Autodesk Inventor part; units mm, degrees
(part 3 of 3)
  line L1861 (14.3835, -12.5591) -> (14.4054, -12.4772)
  line L1862 (17.1782, -13.4855) -> (17.1805, -13.4518)
  line L1863 (17.0231, -13.6469) -> (17.0963, -13.6273)
  line L1864 (17.0963, -13.6273) -> (17.1562, -13.5674)
  line L1865 (17.1562, -13.5674) -> (17.1782, -13.4855)
  line L1866 (6.3458, -17.4083) -> (6.4277, -17.4302)
  line L1867 (6.4277, -17.4302) -> (6.5095, -17.4083)
  line L1868 (6.5095, -17.4083) -> (6.5695, -17.3484)
  line L1869 (6.5695, -17.3484) -> (6.5731, -17.2918)
  line L1870 (1.5112, -17.3523) -> (1.5566, -17.4083)
  line L1871 (1.5566, -17.4083) -> (1.6384, -17.4302)
  line L1872 (1.6384, -17.4302) -> (1.7203, -17.4083)
  line L1873 (1.7203, -17.4083) -> (1.7976, -17.3523)
  line L1874 (-4.3089, -17.3184) -> (-4.3009, -17.3484)
  line L1875 (-4.3009, -17.3484) -> (-4.241, -17.4083)
  line L1876 (-4.241, -17.4083) -> (-4.1591, -17.4302)
  line L1877 (-4.1591, -17.4302) -> (-4.0772, -17.4083)
  line L1878 (-4.0772, -17.4083) -> (-4.049, -17.3801)
  line L1879 (-0.2705, -17.3523) -> (-0.2079, -17.4083)
  line L1880 (-0.2079, -17.4083) -> (-0.126, -17.4302)
  line L1881 (-0.126, -17.4302) -> (-0.0442, -17.4083)
  line L1882 (-0.0442, -17.4083) -> (0.0159, -17.3523)
  line L1883 (-6.0807, -15.5268) -> (-6.0653, -15.5839)
  line L1884 (-6.0653, -15.5839) -> (-6.0054, -15.6438)
  line L1885 (-6.0054, -15.6438) -> (-5.9235, -15.6658)
  line L1886 (-5.9235, -15.6658) -> (-5.8417, -15.6438)
  line L1887 (-5.8417, -15.6438) -> (-5.8234, -15.6256)
  line L1888 (-9.1183, -14.7466) -> (-9.0901, -14.8277)
  line L1889 (-9.0901, -14.8277) -> (-9.0302, -14.8876)
  line L1890 (-9.0302, -14.8876) -> (-8.9483, -14.9096)
  line L1891 (-8.9483, -14.9096) -> (-8.8703, -14.8897)
  line L1892 (-11.8848, -14.7458) -> (-11.8629, -14.8277)
  line L1893 (-11.8629, -14.8277) -> (-11.8029, -14.8876)
  line L1894 (-11.8029, -14.8876) -> (-11.721, -14.9096)
  line L1895 (-11.721, -14.9096) -> (-11.6701, -14.8897)
  line L1896 (-13.6492, -15.7541) -> (-13.6273, -15.836)
  line L1897 (-13.6273, -15.836) -> (-13.5674, -15.8959)
  line L1898 (-13.5674, -15.8959) -> (-13.4855, -15.9178)
  line L1899 (-13.4855, -15.9178) -> (-13.4518, -15.9078)
  line L1900 (-15.1443, -17.1424) -> (-15.1397, -17.2223)
  line L1901 (-15.1397, -17.2223) -> (-15.0798, -17.2823)
  line L1902 (-15.0798, -17.2823) -> (-14.9979, -17.3042)
  line L1903 (-17.435, -14.5971) -> (-17.4302, -14.6198)
  line L1904 (-17.4302, -14.6198) -> (-17.4083, -14.7017)
  line L1905 (-17.4083, -14.7017) -> (-17.3484, -14.7616)
  line L1906 (-17.3484, -14.7616) -> (-17.2747, -14.7813)
  line L1907 (-15.6533, -13.1972) -> (-15.6658, -13.2334)
  line L1908 (-15.6658, -13.2334) -> (-15.6438, -13.3153)
  line L1909 (-15.6438, -13.3153) -> (-15.5839, -13.3752)
  line L1910 (-15.5839, -13.3752) -> (-15.502, -13.3972)
  line L1911 (-15.1443, -11.4156) -> (-15.1616, -11.469)
  line L1912 (-15.1616, -11.469) -> (-15.1397, -11.5509)
  line L1913 (-15.1397, -11.5509) -> (-15.0798, -11.6108)
  line L1914 (-15.0798, -11.6108) -> (-14.9979, -11.6327)
  line L1915 (-14.8897, -8.6158) -> (-14.9096, -8.6963)
  line L1916 (-14.9096, -8.6963) -> (-14.8876, -8.7781)
  line L1917 (-14.8876, -8.7781) -> (-14.8277, -8.8381)
  line L1918 (-14.8277, -8.8381) -> (-14.7466, -8.8638)
  line L1919 (-15.6275, -6.0774) -> (-15.6438, -6.0937)
  line L1920 (-15.6438, -6.0937) -> (-15.6658, -6.1756)
  line L1921 (-15.6658, -6.1756) -> (-15.6438, -6.2575)
  line L1922 (-15.6438, -6.2575) -> (-15.5839, -6.3174)
  line L1923 (-15.5839, -6.3174) -> (-15.5101, -6.3185)
  line L1924 (-17.3801, -4.049) -> (-17.4083, -4.0772)
  line L1925 (-17.4083, -4.0772) -> (-17.4302, -4.1591)
  line L1926 (-17.4302, -4.1591) -> (-17.4083, -4.241)
  line L1927 (-17.4083, -4.241) -> (-17.3484, -4.3009)
  line L1928 (-17.3484, -4.3009) -> (-17.3184, -4.3089)
  line L1929 (-17.3523, -1.5112) -> (-17.4083, -1.5566)
  line L1930 (-17.4083, -1.5566) -> (-17.4302, -1.6384)
  line L1931 (-17.4302, -1.6384) -> (-17.4083, -1.7203)
  line L1932 (-17.4083, -1.7203) -> (-17.3523, -1.7976)
  line L1933 (-17.3523, 1.034) -> (-17.4083, 0.9641)
  line L1934 (-17.4083, 0.9641) -> (-17.4302, 0.8822)
  line L1935 (-17.4302, 0.8822) -> (-17.4083, 0.8004)
  line L1936 (-17.4083, 0.8004) -> (-17.3523, 0.7476)
  line L1937 (-17.3223, 3.8037) -> (-17.3484, 3.7968)
  line L1938 (-17.3484, 3.7968) -> (-17.4083, 3.7368)
  line L1939 (-17.4083, 3.7368) -> (-17.4302, 3.6549)
  line L1940 (-17.4302, 3.6549) -> (-17.4083, 3.5731)
  line L1941 (-17.4083, 3.5731) -> (-17.3762, 3.541)
  line L1942 (-17.2918, 6.8276) -> (-17.3484, 6.8215)
  line L1943 (-17.3484, 6.8215) -> (-17.4083, 6.7616)
  line L1944 (-17.4083, 6.7616) -> (-17.4302, 6.6797)
  line L1945 (-17.4302, 6.6797) -> (-17.4083, 6.5979)
  line L1946 (-17.2918, 9.3729) -> (-17.3484, 9.3422)
  line L1947 (-17.3484, 9.3422) -> (-17.4083, 9.2823)
  line L1948 (-17.4083, 9.2823) -> (-17.4302, 9.2004)
  line L1949 (-17.4302, 9.2004) -> (-17.4117, 9.1311)
  line L1950 (-17.2824, 11.6285) -> (-17.3484, 11.6108)
  line L1951 (-17.3484, 11.6108) -> (-17.4083, 11.5509)
  line L1952 (-17.4083, 11.5509) -> (-17.4302, 11.469)
  line L1953 (-17.4302, 11.469) -> (-17.435, 11.4156)
  line L1954 (-17.0963, 12.8711) -> (-17.1562, 12.8112)
  line L1955 (-15.7541, 13.1451) -> (-15.836, 13.1232)
  line L1956 (-15.836, 13.1232) -> (-15.8959, 13.0632)
  line L1957 (-15.8959, 13.0632) -> (-15.9178, 12.9814)
  line L1958 (-15.9178, 12.9814) -> (-15.9078, 12.9427)
  line L1959 (-13.9608, 17.435) -> (-13.9896, 17.4302)
  line L1960 (-14.0715, 17.4083) -> (-14.1314, 17.3484)
  line L1961 (-12.8112, 17.4083) -> (-12.8711, 17.3484)
  line L1962 (-12.8711, 17.3484) -> (-12.8896, 17.2793)
  line L1963 (-16.2927, 5.5739) -> (-16.3401, 5.5612)
  line L1964 (-16.3401, 5.5612) -> (-16.4, 5.5013)
  line L1965 (-16.4, 5.5013) -> (-16.422, 5.4194)
  line L1966 (-16.422, 5.4194) -> (-16.4, 5.3375)
  line L1967 (-16.4, 5.3375) -> (-16.3795, 5.317)
  line L1968 (-16.01, 11.8838) -> (-16.088, 11.8629)
  line L1969 (-16.088, 11.8629) -> (-16.148, 11.8029)
  line L1970 (-16.148, 11.8029) -> (-16.1699, 11.721)
  line L1971 (-16.1699, 11.721) -> (-16.1624, 11.6701)
  line L1972 (-5.307, 13.9989) -> (-5.3375, 14.0054)
  line L1973 (-5.3375, 14.0054) -> (-5.4194, 14.0273)
  line L1974 (-5.4194, 14.0273) -> (-5.5013, 14.0054)
  line L1975 (-5.5013, 14.0054) -> (-5.5612, 13.9455)
  line L1976 (-5.5612, 13.9455) -> (-5.5789, 13.8796)
  line L1977 (1.034, 17.3523) -> (0.9641, 17.4083)
  line L1978 (0.9641, 17.4083) -> (0.8822, 17.4302)
  line L1979 (0.8822, 17.4302) -> (0.8004, 17.4083)
  line L1980 (0.8004, 17.4083) -> (0.7476, 17.3523)
  line L1981 (7.5912, 16.5282) -> (7.5777, 16.5922)
  line L1982 (7.5777, 16.5922) -> (7.5178, 16.6521)
  line L1983 (7.5178, 16.6521) -> (7.4359, 16.674)
  line L1984 (7.4359, 16.674) -> (7.3541, 16.6521)
  line L1985 (12.4331, 11.7368) -> (12.3512, 11.7588)
  line L1986 (12.3512, 11.7588) -> (12.3175, 11.7497)
  line L1987 (12.5032, 11.5513) -> (12.515, 11.595)
  line L1988 (15.4137, 10.4607) -> (15.3918, 10.5426)
  line L1989 (15.3918, 10.5426) -> (15.3318, 10.6025)
  line L1990 (15.3318, 10.6025) -> (15.25, 10.6245)
  line L1991 (15.3988, 10.3975) -> (15.4137, 10.4607)
  line L1992 (14.4054, 9.7045) -> (14.3835, 9.7864)
  line L1993 (14.3835, 9.7864) -> (14.3236, 9.8463)
  line L1994 (14.3236, 9.8463) -> (14.2375, 9.8819)
  line L1995 (14.3807, 9.6339) -> (14.4054, 9.7045)
  line L1996 (14.1534, 3.6549) -> (14.1314, 3.7368)
  line L1997 (14.1314, 3.7368) -> (14.0715, 3.7968)
  line L1998 (14.0715, 3.7968) -> (14.0202, 3.8105)
  line L1999 (14.0926, 3.5343) -> (14.1314, 3.5731)
  line L2000 (14.1314, 3.5731) -> (14.1534, 3.6549)
  line L2001 (16.1699, -0.6302) -> (16.148, -0.5483)
  line L2002 (16.148, -0.5483) -> (16.0797, -0.4931)
  line L2003 (16.0797, -0.7795) -> (16.148, -0.712)
  line L2004 (16.148, -0.712) -> (16.1699, -0.6302)
  line L2005 (13.6492, -5.9235) -> (13.6273, -5.8417)
  line L2006 (13.6273, -5.8417) -> (13.6171, -5.816)
  line L2007 (13.4947, -6.0848) -> (13.5674, -6.0653)
  line L2008 (13.5674, -6.0653) -> (13.6273, -6.0054)
  line L2009 (13.6273, -6.0054) -> (13.6492, -5.9235)
  line L2010 (14.1534, -7.9401) -> (14.1262, -7.8522)
  line L2011 (13.983, -8.1002) -> (14.0715, -8.0819)
  line L2012 (14.0715, -8.0819) -> (14.1314, -8.0219)
  line L2013 (14.1314, -8.0219) -> (14.1534, -7.9401)
  line L2014 (4.6778, -14.3539) -> (4.7074, -14.3835)
  line L2015 (4.7074, -14.3835) -> (4.7892, -14.4054)
  line L2016 (4.7892, -14.4054) -> (4.8711, -14.3835)
  line L2017 (4.8711, -14.3835) -> (4.9311, -14.3236)
  line L2018 (4.9311, -14.3236) -> (4.9466, -14.2655)
  line L2019 (-1.034, -15.3161) -> (-0.9641, -15.3918)
  line L2020 (-0.9641, -15.3918) -> (-0.8822, -15.4137)
  line L2021 (-0.8822, -15.4137) -> (-0.8004, -15.3918)
  line L2022 (-0.8004, -15.3918) -> (-0.7476, -15.3161)
  line L2023 (-13.0849, 10.6184) -> (-13.1074, 10.6245)
  line L2024 (-13.1074, 10.6245) -> (-13.1893, 10.6025)
  line L2025 (-11.1681, 12.88) -> (-11.2169, 12.8931)
  line L2026 (-11.2169, 12.8931) -> (-11.2988, 12.8711)
  line L2027 (-11.2988, 12.8711) -> (-11.3587, 12.8112)
  line L2028 (-11.3587, 12.8112) -> (-11.3807, 12.7293)
  line L2029 (-11.3807, 12.7293) -> (-11.373, 12.7007)
  line L2030 (-14.2233, 13.3923) -> (-14.2417, 13.3972)
  line L2031 (-14.2417, 13.3972) -> (-14.3236, 13.3752)
  line L2032 (-14.3236, 13.3752) -> (-14.3835, 13.3153)
  line L2033 (-14.3835, 13.3153) -> (-14.4054, 13.2334)
  line L2034 (-14.4054, 13.2334) -> (-14.3807, 13.1972)
  line L2035 (-14.8719, 11.6327) -> (-14.9537, 11.6108)
  line L2036 (-14.9537, 11.6108) -> (-15.0137, 11.5509)
  line L2037 (-15.0137, 11.5509) -> (-15.0356, 11.469)
  line L2038 (-15.0356, 11.469) -> (-15.017, 11.4156)
  line L2039 (-14.8738, 9.3729) -> (-14.9537, 9.3422)
  line L2040 (-14.9537, 9.3422) -> (-15.0137, 9.2823)
  line L2041 (-15.0137, 9.2823) -> (-15.0356, 9.2004)
  line L2042 (-15.0356, 9.2004) -> (-15.017, 9.1248)
  line L2043 (17.4302, 4.5372) -> (17.4083, 4.6191)
  line L2044 (17.4083, 4.6191) -> (17.3484, 4.679)
  line L2045 (17.3484, 4.679) -> (17.3155, 4.6878)
  line L2046 (17.383, 4.43) -> (17.4083, 4.4553)
  line L2047 (17.4083, 4.4553) -> (17.4302, 4.5372)
  line L2048 (17.4302, 1.5124) -> (17.4083, 1.5943)
  line L2049 (17.4083, 1.5943) -> (17.3523, 1.6703)
  line L2050 (17.3523, 1.384) -> (17.4083, 1.4305)
  line L2051 (17.4083, 1.4305) -> (17.4302, 1.5124)
  line L2052 (1.6761, 3.5289) -> (1.6542, 3.6108)
  line L2053 (1.6542, 3.6108) -> (1.5943, 3.6707)
  line L2054 (1.5124, 3.6927) -> (1.4305, 3.6707)
  line L2055 (1.4305, 3.6707) -> (1.384, 3.646)
  line L2056 (1.3706, 3.6108) -> (1.3618, 3.5634)
  line L2057 (1.6703, 3.4807) -> (1.6761, 3.5289)
  line L2058 (5.2051, 0) -> (5.1831, 0.0819)
  line L2059 (5.1831, 0.0819) -> (5.1232, 0.1418)
  line L2060 (5.1232, 0.1418) -> (5.0905, 0.1653)
  line L2061 (5.0413, 0.1637) -> (5.0078, 0.1432)
  line L2062 (5.0078, -0.1432) -> (5.0413, -0.1637)
  line L2063 (5.0905, -0.1653) -> (5.1232, -0.1418)
  line L2064 (5.1232, -0.1418) -> (5.1831, -0.0819)
  line L2065 (5.1831, -0.0819) -> (5.2051, 0)
  line L2066 (3.3146, 1.7645) -> (3.2926, 1.8463)
  line L2067 (3.2926, 1.8463) -> (3.2327, 1.9063)
  line L2068 (3.2327, 1.9063) -> (3.1508, 1.9282)
  line L2069 (3.1508, 1.9282) -> (3.0989, 1.9249)
  line L2070 (3.0689, 1.9063) -> (3.0384, 1.8643)
  line L2071 (3.1816, 1.6163) -> (3.2327, 1.6227)
  line L2072 (3.2642, 1.6385) -> (3.2926, 1.6826)
  line L2073 (3.2926, 1.6826) -> (3.3146, 1.7645)
  line L2074 (16.0192, -9.2456) -> (16.088, -9.2162)
  line L2075 (16.088, -9.2162) -> (16.148, -9.1562)
  line L2076 (16.148, -9.1562) -> (16.1699, -9.0744)
  line L2077 (2.67, 15.934) -> (2.6625, 15.962)
  line L2078 (2.6625, 15.962) -> (2.6025, 16.0219)
  line L2079 (2.6025, 16.0219) -> (2.5207, 16.0439)
  line L2080 (2.5207, 16.0439) -> (2.4388, 16.0219)
  line L2081 (2.4388, 16.0219) -> (2.3951, 15.9783)
  line L2082 (7.0821, 15.7647) -> (7.0736, 15.836)
  line L2083 (7.0736, 15.836) -> (7.0137, 15.8959)
  line L2084 (7.0137, 15.8959) -> (6.9318, 15.9178)
  line L2085 (6.9318, 15.9178) -> (6.8499, 15.8959)
  line L2086 (3.2986, 17.3261) -> (3.2926, 17.3484)
  line L2087 (3.2926, 17.3484) -> (3.2327, 17.4083)
  line L2088 (3.2327, 17.4083) -> (3.1508, 17.4302)
  line L2089 (3.1508, 17.4302) -> (3.0689, 17.4083)
  line L2090 (3.0689, 17.4083) -> (3.0384, 17.3523)
  line L2091 (-4.1616, 12.9808) -> (-4.2032, 12.9971)
  line L2092 (-4.2032, 12.9971) -> (-4.2851, 13.0191)
  line L2093 (-4.4269, 12.9372) -> (-4.4443, 12.8723)
  line L2094 (3.8187, -2.1426) -> (3.7968, -2.0607)
  line L2095 (3.7968, -2.0607) -> (3.7733, -2.0203)
  line L2096 (3.7368, -2.0008) -> (3.6906, -1.9981)
  line L2097 (3.5474, -2.2461) -> (3.5731, -2.2844)
  line L2098 (3.6079, -2.3067) -> (3.6549, -2.3063)
  line L2099 (3.6549, -2.3063) -> (3.7368, -2.2844)
  line L2100 (3.7368, -2.2844) -> (3.7968, -2.2244)
  line L2101 (3.7968, -2.2244) -> (3.8187, -2.1426)
  line L2102 (13.1972, -15.1443) -> (13.2334, -15.1616)
  line L2103 (13.3153, -15.1397) -> (13.3752, -15.0798)
  line L2104 (13.3752, -15.0798) -> (13.3972, -14.9979)
  line L2105 (-1.2345, 8.2721) -> (-1.3045, 8.3339)
  line L2106 (-1.3045, 8.3339) -> (-1.3864, 8.3559)
  line L2107 (-1.3864, 8.3559) -> (-1.4682, 8.3339)
  line L2108 (-1.4682, 8.3339) -> (-1.5282, 8.274)
  line L2109 (-1.5282, 8.274) -> (-1.5431, 8.1894)
  line L2110 (-14.8738, 7.3366) -> (-14.9537, 7.3257)
  line L2111 (-14.9537, 7.3257) -> (-15.0137, 7.2657)
  line L2112 (-15.0137, 7.2657) -> (-15.0356, 7.1839)
  line L2113 (-15.0356, 7.1839) -> (-15.017, 7.0886)
  line L2114 (-14.9015, 4.819) -> (-14.9537, 4.805)
  line L2115 (-14.9537, 4.805) -> (-15.0137, 4.7451)
  line L2116 (-15.0137, 4.7451) -> (-15.0356, 4.6632)
  line L2117 (-15.0356, 4.6632) -> (-15.0137, 4.5813)
  line L2118 (-15.0137, 4.5813) -> (-14.9844, 4.5521)
  line L2119 (-15.3161, -0.4931) -> (-15.3918, -0.5483)
  line L2120 (-15.3918, -0.5483) -> (-15.4137, -0.6302)
  line L2121 (-15.4137, -0.6302) -> (-15.3918, -0.712)
  line L2122 (-15.3918, -0.712) -> (-15.3161, -0.7795)
  line L2123 (13.3972, 2.1426) -> (13.3752, 2.2244)
  line L2124 (13.3752, 2.2244) -> (13.3153, 2.2844)
  line L2125 (13.3153, 2.2844) -> (13.2799, 2.3067)
  line L2126 (13.3232, 2.0087) -> (13.3752, 2.0607)
  line L2127 (13.3752, 2.0607) -> (13.3972, 2.1426)
  line L2128 (14.6356, 2.4765) -> (14.5756, 2.5364)
  line L2129 (14.5756, 2.5364) -> (14.5525, 2.5612)
  line L2130 (-0.7404, 3.7368) -> (-0.8004, 3.7968)
  line L2131 (-0.8004, 3.7968) -> (-0.8822, 3.8187)
  line L2132 (-0.8822, 3.8187) -> (-0.9641, 3.7968)
  line L2133 (-0.9641, 3.7968) -> (-1.024, 3.7368)
  line L2134 (-1.024, 3.7368) -> (-1.046, 3.6549)
  line L2135 (-1.046, 3.6549) -> (-1.034, 3.6079)
  line L2136 (-1.024, 3.5731) -> (-0.9735, 3.5474)
  line L2137 (-0.7476, 3.6079) -> (-0.7185, 3.6549)
  line L2138 (11.1286, -2.1426) -> (11.1067, -2.0607)
  line L2139 (11.1067, -2.0607) -> (11.05, -2.004)
  line L2140 (10.9892, -2.3067) -> (11.0467, -2.2844)
  line L2141 (11.0467, -2.2844) -> (11.1067, -2.2244)
  line L2142 (11.1067, -2.2244) -> (11.1286, -2.1426)
  line L2143 (7.9401, 7.688) -> (7.9063, 7.814)
  line L2144 (7.9063, 7.814) -> (7.814, 7.9063)
  line L2145 (7.814, 7.9063) -> (7.688, 7.9401)
  line L2146 (7.688, 7.9401) -> (7.562, 7.9063)
  line L2147 (7.562, 7.9063) -> (7.5426, 7.8903)
  line L2148 (7.8903, 7.5426) -> (7.9063, 7.562)
  line L2149 (7.9063, 7.562) -> (7.9401, 7.688)
  line L2150 (-7.5426, 7.8903) -> (-7.562, 7.9063)
  line L2151 (-7.562, 7.9063) -> (-7.688, 7.9401)
  line L2152 (-7.688, 7.9401) -> (-7.814, 7.9063)
  line L2153 (-7.814, 7.9063) -> (-7.9063, 7.814)
  line L2154 (-7.9063, 7.814) -> (-7.9401, 7.688)
  line L2155 (-7.9401, 7.688) -> (-7.9063, 7.562)
  line L2156 (-7.9063, 7.562) -> (-7.8903, 7.5426)
  line L2157 (7.9401, -7.688) -> (7.9063, -7.562)
  line L2158 (7.9063, -7.562) -> (7.8903, -7.5426)
  line L2159 (7.5426, -7.8903) -> (7.562, -7.9063)
  line L2160 (7.562, -7.9063) -> (7.688, -7.9401)
  line L2161 (7.688, -7.9401) -> (7.814, -7.9063)
  line L2162 (7.814, -7.9063) -> (7.9063, -7.814)
  line L2163 (7.9063, -7.814) -> (7.9401, -7.688)
  line L2164 (-14.058, 14.7625) -> (-13.9246, 14.6291)
  line L2165 (8.7971, -13.789) -> (8.7521, -13.7185)
  line L2166 (-8.1218, 18.4531) -> (-8.0433, 18.2747)
  line L2167 (1.384, 3.646) -> (1.3706, 3.6108)
  line L2168 (1.8709, 12.8535) -> (1.8806, 12.8171)
  line L2169 (1.8806, 12.8171) -> (1.893, 12.7709)
  line L2170 (-17.4429, -13.6053) -> (-17.2743, -13.4738)
  line L2171 (-17.7589, -13.846) -> (-17.5873, -13.7121)
  line L2172 (-13.9642, -17.5873) -> (-14.1005, -17.7589)
  line L2173 (-17.0151, 12.8535) -> (-17.025, 12.8902)
  line L2174 (-17.025, 12.8902) -> (-17.0373, 12.9362)
  line L2175 (10.5628, 15.2335) -> (10.6245, 15.25)
  line L2176 (10.6245, 15.25) -> (10.6455, 15.2556)
  line L2177 (-6.6336, 14.1708) -> (-6.5887, 14.1259)
  line L2178 (-6.5887, 14.1259) -> (-6.5731, 14.1102)
  line L2179 (-6.3251, 14.2534) -> (-6.3458, 14.2575)
  line L2180 (-6.3458, 14.2575) -> (-6.3472, 14.3361)
  line L2181 (11.5809, 14.2154) -> (11.6327, 14.2417)
  line L2182 (11.6327, 14.2417) -> (11.6636, 14.2375)
  line L2183 (-7.9063, -7.562) -> (-7.9835, -7.6358)
  line L2184 (16.8433, 6.9835) -> (16.9042, 6.976)
  line L2185 (16.9042, 6.976) -> (16.9259, 6.9614)
  line L2186 (12.3286, 13.5725) -> (12.3126, 13.5129)
  line L2187 (12.3126, 13.5129) -> (12.3064, 13.4899)
  line L2188 (12.4718, 13.3245) -> (12.5082, 13.3343)
  line L2189 (12.5082, 13.3343) -> (12.5544, 13.3467)
  line L2190 (13.3467, 12.5544) -> (13.3343, 12.5082)
  line L2191 (13.3343, 12.5082) -> (13.3245, 12.4718)
  line L2192 (13.4899, 12.3064) -> (13.5129, 12.3126)
  line L2193 (13.5129, 12.3126) -> (13.5725, 12.3286)
  line L2194 (4.5369, 17.2918) -> (4.5615, 17.3164)
  line L2195 (4.5615, 17.3164) -> (4.5974, 17.3523)
  line L2196 (6.8341, 15.9078) -> (6.8499, 15.8959)
  line L2197 (6.8499, 15.8959) -> (6.8563, 15.8252)
  line L2198 (4.2889, 17.435) -> (4.303, 17.3821)
  line L2199 (4.303, 17.3821) -> (4.311, 17.3523)
  line L2200 (14.359, 11.5435) -> (14.3677, 11.5067)
  line L2201 (14.3677, 11.5067) -> (14.3426, 11.4536)
  line L2202 (-7.6358, -7.9835) -> (-7.562, -7.9063)
  line L2203 (8.1067, 17.435) -> (8.1137, 17.4092)
  line L2204 (8.1137, 17.4092) -> (8.1289, 17.3523)
  line L2205 (5.4342, 17.435) -> (5.4461, 17.3908)
  line L2206 (5.4461, 17.3908) -> (5.4564, 17.3523)
  line L2207 (5.6822, 17.2918) -> (5.6981, 17.3077)
  line L2208 (5.6981, 17.3077) -> (5.7428, 17.3523)
  line L2209 (6.5796, 17.435) -> (6.5979, 17.4083)
  line L2210 (6.5979, 17.4083) -> (6.6017, 17.3523)
  line L2211 (17.3523, 7.8744) -> (17.4086, 7.8593)
  line L2212 (17.4086, 7.8593) -> (17.435, 7.8522)
  line L2213 (12.3286, 11.7908) -> (12.3175, 11.7497)
  line L2214 (12.3175, 11.7497) -> (12.3064, 11.7082)
  line L2215 (12.4718, 11.5428) -> (12.5032, 11.5513)
  line L2216 (12.5032, 11.5513) -> (12.5544, 11.565)
  line L2217 (3.0162, 15.3988) -> (3.0289, 15.3517)
  line L2218 (3.0289, 15.3517) -> (3.0384, 15.3161)
  line L2219 (15.2556, 10.6455) -> (15.25, 10.6245)
  line L2220 (15.25, 10.6245) -> (15.2335, 10.5628)
  line L2221 (2.2461, 16.7828) -> (2.2844, 16.8442)
  line L2222 (2.2844, 16.8442) -> (2.3067, 16.8433)
  line L2223 (17.3523, 5.8382) -> (17.3937, 5.8271)
  line L2224 (17.3937, 5.8271) -> (17.435, 5.816)
  line L2225 (14.2542, -4.2864) -> (14.2247, -4.2965)
  line L2226 (14.2247, -4.2965) -> (14.1708, -4.311)
  line L2227 (14.1102, -4.5369) -> (14.1414, -4.568)
  line L2228 (14.1414, -4.568) -> (14.1708, -4.5974)
  line L2229 (17.3077, -10.3975) -> (17.2886, -10.4026)
  line L2230 (17.2886, -10.4026) -> (17.2251, -10.4196)
  line L2231 (17.1424, -10.5628) -> (17.1577, -10.6198)
  line L2232 (17.1577, -10.6198) -> (17.1645, -10.6455)
  line L2233 (13.341, 10.7798) -> (13.3392, 10.7451)
  line L2234 (13.3392, 10.7451) -> (13.3245, 10.6901)
  line L2235 (14.2154, -10.8173) -> (14.2417, -10.8765)
  line L2236 (14.2417, -10.8765) -> (14.2375, -10.9)
  line L2237 (-1.893, 12.7709) -> (-1.8806, 12.8171)
  line L2238 (-1.8806, 12.8171) -> (-1.8709, 12.8535)
  line L2239 (16.7606, -12.09) -> (16.7724, -12.1342)
  line L2240 (16.7724, -12.1342) -> (16.7828, -12.1726)
  line L2241 (17.0151, -13.6171) -> (17.0231, -13.6469)
  line L2242 (17.0231, -13.6469) -> (17.0373, -13.6998)
  line L2243 (11.1651, -15.2479) -> (11.1286, -15.25)
  line L2244 (11.1286, -15.25) -> (11.0719, -15.2335)
  line L2245 (12.1791, -12.3445) -> (12.1884, -12.3791)
  line L2246 (12.1884, -12.3791) -> (12.2013, -12.4272)
  line L2247 (13.4453, -17.2918) -> (13.3941, -17.2781)
  line L2248 (13.3941, -17.2781) -> (13.3626, -17.2697)
  line L2249 (12.4272, -12.2013) -> (12.3791, -12.1884)
  line L2250 (12.3791, -12.1884) -> (12.3445, -12.1791)
  line L2251 (11.1696, -17.282) -> (11.124, -17.2836)
  line L2252 (11.124, -17.2836) -> (11.0719, -17.2697)
  line L2253 (10.9287, -17.3523) -> (10.9116, -17.416)
  line L2254 (10.9116, -17.416) -> (10.9065, -17.435)
  line L2255 (8.6379, -17.3523) -> (8.6224, -17.4104)
  line L2256 (8.6224, -17.4104) -> (8.6158, -17.435)
  line L2257 (-2.2748, 14.6798) -> (-2.2655, 14.7144)
  line L2258 (-2.2655, 14.7144) -> (-2.2527, 14.7625)
  line L2259 (4.0883, -17.3523) -> (4.0563, -17.3203)
  line L2260 (4.0563, -17.3203) -> (4.0278, -17.2918)
  line L2261 (3.802, -17.3523) -> (3.795, -17.3782)
  line L2262 (3.795, -17.3782) -> (3.7798, -17.435)
  line L2263 (-13.579, 16.5229) -> (-13.522, 16.5147)
  line L2264 (-13.522, 16.5147) -> (-13.4899, 16.5061)
  line L2265 (-4.0343, -17.435) -> (-4.049, -17.3801)
  line L2266 (-4.049, -17.3801) -> (-4.0565, -17.3523)
  line L2267 (-4.2823, -17.2918) -> (-4.3089, -17.3184)
  line L2268 (-4.3089, -17.3184) -> (-4.3429, -17.3523)
  line L2269 (-13.4899, -13.3245) -> (-13.5157, -13.3314)
  line L2270 (-13.5157, -13.3314) -> (-13.5725, -13.3467)
  line L2271 (-1.9916, -17.2918) -> (-2.0323, -17.3484)
  line L2272 (-2.0323, -17.3484) -> (-2.0521, -17.3523)
  line L2273 (-2.8379, 3.6906) -> (-2.8104, 3.6549)
  line L2274 (-8.8925, 17.3523) -> (-8.8767, 17.411)
  line L2275 (-8.8767, 17.411) -> (-8.8703, 17.435)
  line L2276 (-14.9979, 16.3752) -> (-15.1443, 16.535)
  line L2277 (15.1443, -1.9089) -> (15.1055, -1.9193)
  line L2278 (15.1055, -1.9193) -> (14.6352, -2.0453)
  line L2279 (16.535, -15.1443) -> (16.3752, -14.9979)
  line L2280 (-13.7258, -17.2743) -> (-13.8598, -17.4429)
  line L2281 (18.2747, -8.2953) -> (18.4531, -8.3763)
  line L2282 (4.0815, 16.1624) -> (4.0421, 16.0062)
  line L2283 (-15.3988, -16.535) -> (-15.25, -16.3752)
  line L2284 (-16.6273, -14.9979) -> (-16.7895, -15.1443)
  line L2285 (14.9979, -16.3752) -> (15.1443, -16.535)
  line L2286 (-14.2088, 17.2918) -> (-14.1508, 17.2762)
  line L2287 (-14.1508, 17.2762) -> (-14.1262, 17.2697)
  line L2288 (-11.9181, 17.2918) -> (-11.8807, 17.2818)
  line L2289 (-11.8807, 17.2818) -> (-11.8354, 17.2697)
  line L2290 (5.9235, 15.502) -> (5.9813, 15.6533)
  line L2291 (-16.535, 15.1443) -> (-16.3752, 14.9979)
  line L2292 (14.9979, -3.907) -> (15.1443, -3.9451)
  line L2293 (-13.2334, 15.3085) -> (-13.3626, 15.4579)
  line L2294 (-8.0176, 16.0351) -> (-8.0567, 16.1813)
  line L2295 (-8.0567, 16.1813) -> (-8.0858, 16.2896)
  line L2296 (-8.9675, 15.7806) -> (-8.9049, 15.718)
  line L2297 (-8.9049, 15.718) -> (-8.7811, 15.5943)
  line L2298 (-8.0176, 13.9989) -> (-8.0639, 14.172)
  line L2299 (-8.0639, 14.172) -> (-8.0858, 14.2534)
  line L2300 (-8.9675, 13.7444) -> (-8.8977, 13.6746)
  line L2301 (-8.8977, 13.6746) -> (-8.7811, 13.5581)
  line L2302 (-12.4337, 13.1081) -> (-12.441, 13.1354)
  line L2303 (-12.441, 13.1354) -> (-12.4558, 13.1907)
  line L2304 (-12.6817, 12.9649) -> (-12.6331, 12.9518)
  line L2305 (-12.6331, 12.9518) -> (-12.599, 12.9427)
  line L2306 (-0.9925, 5.7533) -> (-1.0022, 5.8095)
  line L2307 (11.3264, 12.6882) -> (11.373, 12.7007)
  line L2308 (11.373, 12.7007) -> (11.4091, 12.7103)
  line L2309 (11.1832, 12.9362) -> (11.1681, 12.88)
  line L2310 (11.1681, 12.88) -> (11.161, 12.8535)
  line L2311 (10.6245, 13.2334) -> (10.6455, 13.2194)
  line L2312 (14.2154, -12.599) -> (14.2417, -12.641)
  line L2313 (14.2417, -12.641) -> (14.2375, -12.6817)
  line L2314 (6.3472, -17.3523) -> (6.3458, -17.4083)
  line L2315 (6.3458, -17.4083) -> (6.3251, -17.435)
  line L2316 (-5.816, -15.6533) -> (-5.8234, -15.6256)
  line L2317 (-5.8234, -15.6256) -> (-5.8382, -15.5706)
  line L2318 (-6.064, -15.5101) -> (-6.0807, -15.5268)
  line L2319 (-6.0807, -15.5268) -> (-6.1245, -15.5706)
  line L2320 (-11.8354, -14.7244) -> (-11.8848, -14.7458)
  line L2321 (-11.8848, -14.7458) -> (-11.9181, -14.7466)
  line L2322 (-13.6171, -15.7425) -> (-13.6492, -15.7541)
  line L2323 (-13.6492, -15.7541) -> (-13.6998, -15.7647)
  line L2324 (-14.9789, -17.3077) -> (-14.9979, -17.3042)
  line L2325 (-14.9979, -17.3042) -> (-15.0011, -17.2251)
  line L2326 (-17.2918, -14.8452) -> (-17.2747, -14.7813)
  line L2327 (-17.2747, -14.7813) -> (-17.2697, -14.7625)
  line L2328 (-15.5101, -13.4453) -> (-15.502, -13.3972)
  line L2329 (-15.502, -13.3972) -> (-15.488, -13.3626)
  line L2330 (-15.0011, -11.6636) -> (-14.9979, -11.6327)
  line L2331 (-14.9979, -11.6327) -> (-14.9789, -11.5809)
  line L2332 (-15.5706, -6.0927) -> (-15.6275, -6.0774)
  line L2333 (-15.6275, -6.0774) -> (-15.6533, -6.0705)
  line L2334 (-17.3523, -4.3429) -> (-17.3184, -4.3089)
  line L2335 (-17.3184, -4.3089) -> (-17.2918, -4.2823)
  line L2336 (-17.3523, -4.0565) -> (-17.3801, -4.049)
  line L2337 (-17.3801, -4.049) -> (-17.435, -4.0343)
  line L2338 (-17.435, 3.5253) -> (-17.3762, 3.541)
  line L2339 (-17.3762, 3.541) -> (-17.3523, 3.5474)
  line L2340 (-17.2918, 3.7733) -> (-17.3223, 3.8037)
  line L2341 (-17.3223, 3.8037) -> (-17.3523, 3.8338)
  line L2342 (-17.435, 6.5796) -> (-17.4083, 6.5979)
  line L2343 (-17.4083, 6.5979) -> (-17.3523, 6.6017)
  line L2344 (-17.435, 9.1248) -> (-17.4117, 9.1311)
  line L2345 (-17.4117, 9.1311) -> (-17.3523, 9.147)
  line L2346 (-17.2697, 11.5809) -> (-17.2824, 11.6285)
  line L2347 (-17.2824, 11.6285) -> (-17.2918, 11.6636)
  line L2348 (-15.7425, 13.1081) -> (-15.7541, 13.1451)
  line L2349 (-15.7541, 13.1451) -> (-15.7647, 13.1907)
  line L2350 (-12.9362, 17.2918) -> (-12.8896, 17.2793)
  line L2351 (-12.8896, 17.2793) -> (-12.8535, 17.2697)
  line L2352 (-16.4169, 5.307) -> (-16.3795, 5.317)
  line L2353 (-16.3795, 5.317) -> (-16.3342, 5.3291)
  line L2354 (-16.2737, 5.555) -> (-16.2927, 5.5739)
  line L2355 (-16.2927, 5.5739) -> (-16.3342, 5.6155)
  line L2356 (-15.997, 11.8354) -> (-16.01, 11.8838)
  line L2357 (-16.01, 11.8838) -> (-16.0192, 11.9181)
  line L2358 (-5.6155, 13.9162) -> (-5.5789, 13.8796)
  line L2359 (-5.5789, 13.8796) -> (-5.555, 13.8557)
  line L2360 (7.3432, 16.6714) -> (7.3541, 16.6521)
  line L2361 (7.3541, 16.6521) -> (7.3653, 16.5888)
  line L2362 (3.2642, 15.2556) -> (3.3027, 15.2941)
  line L2363 (3.3027, 15.2941) -> (3.3248, 15.3161)
  line L2364 (14.0435, 3.5474) -> (14.0926, 3.5343)
  line L2365 (14.0926, 3.5343) -> (14.1262, 3.5253)
  line L2366 (14.0435, 3.8338) -> (14.0202, 3.8105)
  line L2367 (14.0202, 3.8105) -> (13.983, 3.7733)
  line L2368 (12.5163, 2.9111) -> (12.5723, 2.8961)
  line L2369 (12.5723, 2.8961) -> (12.599, 2.889)
  line L2370 (13.4739, -6.064) -> (13.4947, -6.0848)
  line L2371 (13.4947, -6.0848) -> (13.5344, -6.1245)
  line L2372 (4.6928, -14.298) -> (4.6778, -14.3539)
  line L2373 (4.6778, -14.3539) -> (4.6706, -14.3807)
  line L2374 (4.9792, -14.298) -> (4.9466, -14.2655)
  line L2375 (4.9466, -14.2655) -> (4.9187, -14.2375)
  line L2376 (-13.3467, -13.5725) -> (-13.3314, -13.5157)
  line L2377 (-13.3314, -13.5157) -> (-13.3245, -13.4899)
  line L2378 (-13.07, 10.5628) -> (-13.0849, 10.6184)
  line L2379 (-13.0849, 10.6184) -> (-13.0921, 10.6455)
  line L2380 (-11.161, 12.8535) -> (-11.1681, 12.88)
  line L2381 (-11.1681, 12.88) -> (-11.1832, 12.9362)
  line L2382 (-11.4091, 12.7103) -> (-11.373, 12.7007)
  line L2383 (-11.373, 12.7007) -> (-11.3264, 12.6882)
  line L2384 (-14.2154, 13.3626) -> (-14.2417, 13.3972)
  line L2385 (-14.2417, 13.3972) -> (-14.2375, 13.4453)
  line L2386 (-14.8517, 11.5809) -> (-14.8719, 11.6327)
  line L2387 (-14.8719, 11.6327) -> (-14.8738, 11.6636)
  line L2388 (17.3523, 4.4383) -> (17.383, 4.43)
  line L2389 (17.383, 4.43) -> (17.435, 4.4161)
  line L2390 (17.3523, 4.7246) -> (17.3155, 4.6878)
  line L2391 (17.3155, 4.6878) -> (17.2918, 4.6641)
  line L2392 (1.6761, 3.5289) -> (1.6925, 3.5634)
  line L2393 (1.6542, 3.447) -> (1.6703, 3.4807)
  line L2394 (1.4445, 3.7065) -> (1.4305, 3.6707)
  line L2395 (5.1232, -0.1418) -> (5.1732, -0.1432)
  line L2396 (5.0413, -0.1637) -> (5.0905, -0.1653)
  line L2397 (5.0905, 0.1653) -> (5.0413, 0.1637)
  line L2398 (5.1732, 0.1432) -> (5.1232, 0.1418)
  line L2399 (3.2926, 1.6826) -> (3.3248, 1.699)
  line L2400 (3.2327, 1.6227) -> (3.2642, 1.6385)
  line L2401 (3.0989, 1.9249) -> (3.0689, 1.9063)
  line L2402 (3.1816, 1.947) -> (3.1508, 1.9282)
  line L2403 (2.6279, 15.8919) -> (2.67, 15.934)
  line L2404 (2.67, 15.934) -> (2.6884, 15.9524)
  line L2405 (2.3799, 16.0351) -> (2.3951, 15.9783)
  line L2406 (2.3951, 15.9783) -> (2.4021, 15.9524)
  line L2407 (3.2642, 17.2918) -> (3.2986, 17.3261)
  line L2408 (3.2986, 17.3261) -> (3.3248, 17.3523)
  line L2409 (-4.4701, 12.8981) -> (-4.4443, 12.8723)
  line L2410 (-4.4443, 12.8723) -> (-4.4096, 12.8376)
  line L2411 (3.6549, -2.3063) -> (3.6906, -2.3288)
  line L2412 (3.5731, -2.2844) -> (3.6079, -2.3067)
  line L2413 (3.7733, -2.0203) -> (3.7368, -2.0008)
  line L2414 (3.8338, -2.0808) -> (3.7968, -2.0607)
  line L2415 (13.4453, -15.0011) -> (13.3972, -14.9979)
  line L2416 (13.3972, -14.9979) -> (13.3626, -14.9789)
  line L2417 (-15.017, 4.5434) -> (-14.9844, 4.5521)
  line L2418 (-14.9844, 4.5521) -> (-14.9343, 4.5655)
  line L2419 (-14.8738, 4.7914) -> (-14.9015, 4.819)
  line L2420 (-14.9015, 4.819) -> (-14.9343, 4.8519)
  line L2421 (13.2799, 2.0203) -> (13.3232, 2.0087)
  line L2422 (13.3232, 2.0087) -> (13.3626, 1.9981)
  line L2423 (14.5525, 2.2748) -> (14.5881, 2.2653)
  line L2424 (14.5881, 2.2653) -> (14.6352, 2.2527)
  line L2425 (-2.5648, 3.7968) -> (-2.5898, 3.8338)
  line L2426 (-0.7404, 3.7368) -> (-0.7476, 3.7733)
  line L2427 (-1.034, 3.6079) -> (-1.024, 3.5731)
  line L2428 (-1.0562, 3.6906) -> (-1.046, 3.6549)
  line L2429 (11.0719, -1.9981) -> (11.05, -2.004)
  line L2430 (11.05, -2.004) -> (10.9892, -2.0203)
  line L2431 (7.9063, 7.562) -> (7.9835, 7.6358)
  line L2432 (7.6358, 7.9835) -> (7.562, 7.9063)
  line L2433 (-7.9835, 7.6358) -> (-7.9063, 7.562)
  line L2434 (-7.562, 7.9063) -> (-7.6358, 7.9835)
  line L2435 (7.562, -7.9063) -> (7.6358, -7.9835)
  line L2436 (7.9835, -7.6358) -> (7.9063, -7.562)
  line L2437 (10.5628, 13.1972) -> (10.6188, 13.2122)
  line L2438 (-18.4531, -14.2304) -> (-18.4528, -14.5799)
  line L2439 (-2.5648, 3.7968) -> (-2.5049, 3.7368)
  line L2440 (-0.7404, 3.7368) -> (-0.7185, 3.6549)
  dimension "d0" = 36.9062
  constraints: 4882 end point
  measures "d0" distance between parallel lines of L793 L27
extrude "Extrusion1" add sketch "PCB" along normal blind 0.6604 contours L759 L762 L761 L760 L764 L763 L769 L783 L781 L1 L779 L778 L772 L771 L770 L768 L766 L777 L776 L775 L790 L789 L788 L785 L765 L856 L858 L860 L861 L862 L863 L864 L865 L866 L868 L869 L870 L871 L872 L873 L874 L875 L876 L733 L877 L1785 L2280 L83 L2172 L81 L79 L78 L76 L75 L74 L73 L72 L71 L70 L69 L68 L66 L65 L64 L63 L62 L61 L59 L58 L57 L56 L54 L53 L51 L50 L2438 L48 L45 L2171 L44 L2170 L43 L41 L40 L39 L38 L37 L36 L34 L21 L20 L16 L15 L13 L11 L9 L24 L33 L32 L30 L29 L28 L27 L851 L850 L849 L848 L847 L846 L845 L844 L843 L842 L841 L840 L839 L838 L837 L836 L834 L833 L832 L831 L830 L829 L827 L824 L823 L2166 L1783 L910 L911 L913 L914 L915 L916 L917 L920 L921 L922 L923 L924 L925 L927 L928 L930 L931 L932 L933 L934 L935 L936 L937 L822 L821 L819 L818 L817 L816 L815 L814 L813 L812 L811 L810 L809 L808 L807 L806 L804 L803 L802 L801 L800 L799 L796 L795 L757 L793 L878 L881 L882 L884 L885 L887 L888 L889 L890 L891 L892 L893 L894 L895 L896 L898 L899 L900 L902 L903 L904 L906 L908 L1784 L2281 L0
move or copy body "Move Body1" bodies to move or copy 1 copy no rotation origin (0, 0, 0) rotation axis (-0.5773503, -0.5773503, 0.5773503) rotation angle -120
sketch "Sketch3" plane through (-6.6988, 0, 18.4531) normal (0, 1, 0) x (1, 0, 0)
  line L0 (25.1115, 36.8748) -> (25.1115, 0.0244) construction
  line L1 (25.1115, 0.0244) -> (-11.739, 0.0244) construction
  line L2 (-11.739, 0.0244) -> (-11.739, 36.8748) construction
  line L3 (-11.739, 36.8748) -> (25.1115, 36.8748) construction
  point P0 (6.6988, 18.4531)
  constraints: 2 other
decal "Decal1"
sketch "Sketch4" plane through (-6.6988, -0.6604, 18.4531) normal (0, -1, 0) x (1, 0, 0)
  line L0 (25.1191, 0.0337) -> (25.1191, -36.8168) construction
  line L1 (25.1191, -36.8168) -> (-11.7314, -36.8168) construction
  line L2 (-11.7314, -36.8168) -> (-11.7314, 0.0337) construction
  line L3 (-11.7314, 0.0337) -> (25.1191, 0.0337) construction
  point P0 (6.6988, -18.4531)
  constraints: 2 other
decal "Decal2"
body "Solid1"
